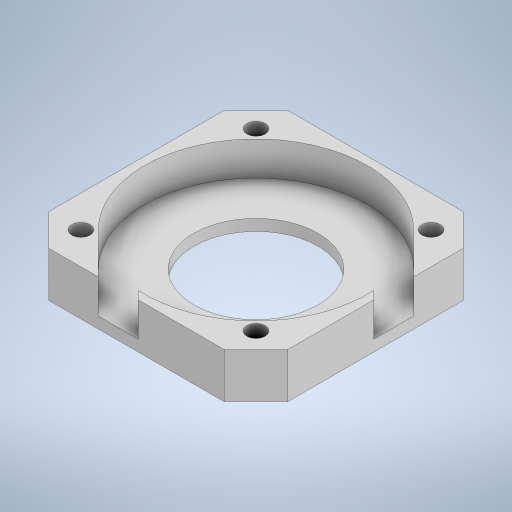
# Autodesk Inventor part: Pumphousing
Saved by Autodesk Inventor 2023 (Build 270158000, 158)
## iProperties
Created: 2022-12-06
Part Number: Pumphousing
Material: Generic
Document SubType Name: Modeling
Designer: Owner
Density: 1 g/cm^3
Appearance: Default
Author: Owner
Autodesk Inventor part; units mm, degrees
ref_plane "YZ Plane" through (0, 0, 0) normal (1, 0, 0) x (0, 1, 0)
ref_plane "XZ Plane" through (0, 0, 0) normal (0, 1, 0) x (-1, 0, 0)
ref_plane "XY Plane" through (0, 0, 0) normal (0, 0, 1) x (1, 0, 0)
sketch "Sketch1" plane through (0, 0, 0) normal (0, 1, 0) x (-1, 0, 0)
  line L0 (-15.5, 21.15) -> (15.5, 21.15)
  line L1 (21.15, 15.5) -> (21.15, -15.5)
  line L2 (15.5, -21.15) -> (-15.5, -21.15)
  line L3 (-21.15, -15.5) -> (-21.15, 15.5)
  line L4 (-21.15, 21.15) -> (21.15, -21.15) construction
  line L5 (21.15, 21.15) -> (-21.15, -21.15) construction
  line L6 (-15.5, 15.5) -> (15.5, 15.5)
  line L7 (15.5, 15.5) -> (15.5, -15.5)
  line L8 (15.5, -15.5) -> (-15.5, -15.5)
  line L9 (-15.5, -15.5) -> (-15.5, 15.5)
  line L10 (-15.5, 15.5) -> (15.5, -15.5) construction
  line L11 (15.5, 15.5) -> (-15.5, -15.5) construction
  circle A0 centre (0, 0) radius 11
  circle A1 centre (15.5, 15.5) radius 1.625
  circle A2 centre (15.5, -15.5) radius 1.625
  circle A3 centre (-15.5, -15.5) radius 1.625
  circle A4 centre (-15.5, 15.5) radius 1.625
  line L12 (15.5, -15.5) -> (15.5, -21.15)
  line L13 (21.15, -15.5) -> (15.5, -21.15)
  line L14 (-15.5, -21.15) -> (-21.15, -15.5)
  line L15 (-21.15, 15.5) -> (-15.5, 21.15)
  line L16 (15.5, 21.15) -> (21.15, 15.5)
  line L17 (0, -15.5) -> (0, -21.15)
  line L18 (0, -15.5) -> (0, -18.325)
  line L19 (0, -18.325) -> (0, -21.15)
  circle A5 centre (0, 0) radius 19.7375
  dimension "d0" = 42.3
  dimension "d1" = 42.3
  dimension "d2" = 31
  dimension "d3" = 31
  dimension "d4" = 22
  dimension "d5" = 3.25
  dimension "d6" = 3.25
  dimension "d7" = 3.25
  dimension "d8" = 3.25
  constraints: 40 end point, 7 midpoint, 6 centre point, 6 coincident, 6 perpendicular, 4 parallel, 3 point on line, 2 horizontal, 1 collinear
  measures "d0" distance of L4.end L5.end
  measures "d1" distance of L5.start L4.end
  measures "d2" distance of L7.end L8.end
  measures "d3" distance of L6.end L7.end
  measures "d4" diameter of A0
  measures "d5" diameter of A1
  measures "d6" diameter of A2
  measures "d7" diameter of A3
  measures "d8" diameter of A4
extrude "Extrusion1" add sketch "Sketch1" along normal blind 2 contours L0 L16 L1 L13 L12 A2 L7 A5 A1 L6 A4 L9 A3 L8 L17 L2 L14 L3 L15 | L2 L17 A5 L8 A2 L12 | A5 L8 L17 | L17 L8 A5 | L8 A5 L7 A2 | A5 L9 L6 L7 L8 | L8 A3 L9 A5 | A5 L9 | L7 A5 | L9 A4 L6 A5 | A5 L6 A1 L7 | A5 L6
sketch "Sketch2" plane through (0, 2, 0) normal (0, 1, 0) x (1, 0, 0)
  line L0 (-15.5, 21.15) -> (15.5, 21.15)
  line L1 (21.15, 15.5) -> (21.15, -15.5)
  line L2 (15.5, -21.15) -> (-15.5, -21.15)
  line L3 (-21.15, -15.5) -> (-21.15, 15.5)
  line L4 (-21.15, 21.15) -> (21.15, -21.15) construction
  line L5 (21.15, 21.15) -> (-21.15, -21.15) construction
  line L6 (-15.5, 15.5) -> (15.5, 15.5)
  line L7 (15.5, 15.5) -> (15.5, -15.5)
  line L8 (15.5, -15.5) -> (-15.5, -15.5)
  line L9 (-15.5, -15.5) -> (-15.5, 15.5)
  line L10 (-15.5, 15.5) -> (15.5, -15.5) construction
  line L11 (15.5, 15.5) -> (-15.5, -15.5) construction
  circle A0 centre (0, 0) radius 11
  circle A1 centre (15.5, 15.5) radius 1.625
  circle A2 centre (15.5, -15.5) radius 1.625
  circle A3 centre (-15.5, -15.5) radius 1.625
  circle A4 centre (-15.5, 15.5) radius 1.625
  line L12 (15.5, -15.5) -> (15.5, -21.15)
  line L13 (21.15, -15.5) -> (15.5, -21.15)
  line L14 (-15.5, -21.15) -> (-21.15, -15.5)
  line L15 (-21.15, 15.5) -> (-15.5, 21.15)
  line L16 (15.5, 21.15) -> (21.15, 15.5)
  line L17 (0, -15.5) -> (0, -21.15)
  line L18 (0, -15.5) -> (0, -18.325)
  line L19 (0, -18.325) -> (0, -21.15)
  circle A5 centre (0, 0) radius 19.7375
  circle A6 centre (0, 0) radius 11 projected
  line L20 (-15.5, -21.15) -> (15.5, -21.15) projected
  line L21 (-13.9565, -13.9565) -> (-6.763, -21.15)
  line L22 (0, 0) -> (7.7782, -7.7782) construction
  line L23 (13.9565, 13.9565) -> (21.15, 6.763)
  circle A7 centre (0, 0) radius 14.7375 construction
  line L24 (-1.1373, -19.7047) -> (0.308, -21.15)
  line L25 (19.7047, 1.1373) -> (21.15, -0.308)
  point P0 (-10.421, -10.421)
  point P1 (10.421, 10.421)
  point P2 (20.4274, 0.4146)
  point P3 (15.5, 12.2196)
  point P4 (15.5, 12.413)
  point P5 (-12.413, -15.5)
  point P6 (-12.2196, -15.5)
  point P7 (0, -20.842)
  point P8 (21.15, -0.308)
  dimension "d15" = 22
  dimension "d11" = 42.3
  dimension "d12" = 42.3
  dimension "d13" = 31
  dimension "d14" = 31
  dimension "d16" = 3.25
  dimension "d17" = 3.25
  dimension "d18" = 3.25
  dimension "d19" = 3.25
  dimension "d23" = 5
  dimension "d24" = 5
  constraints: 50 end point, 8 midpoint, 8 point on line, 7 perpendicular, 6 coincident, 5 centre point, 4 parallel, 4 symmetric about line, 3 point on circle, 2 horizontal, 1 collinear, 7 other
  measures "d11" distance of L4.end L5.end
  measures "d12" distance of L5.start L4.end
  measures "d13" distance of L7.end L8.end
  measures "d14" distance of L6.end L7.end
  measures "d16" diameter of A1
  measures "d17" diameter of A2
  measures "d18" diameter of A3
  measures "d19" diameter of A4
  measures "d24" distance from line of point (20.427, 0.415) L23
extrude "Extrusion2" add sketch "Sketch2" along normal blind 6 contours L0 L16 L1 L23 L7 A1 L6 A5 A4 L9 A3 L8 L21 L2 L14 L3 L15 | L1 L13 L12 A2 L7 A5 L25 | L23 A5 L6 A1 L7 | L8 A3 L9 A5 L21 | L2 L24 L17 A5 L8 A2 L12 | L7 A2 L8 A5 | L24 A5 L17 | A5 L9 A4 L6
body "Solid1"
